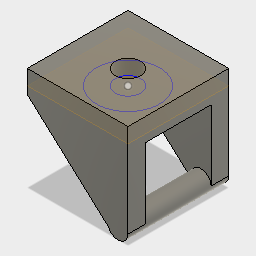
CasterWheelAngle (Autodesk Fusion 360 design; units mm, degrees)
Autodesk Fusion 360 part; units mm, degrees
sketch "Sketch1" plane through (0, 0, 0) normal (0, 1, 0) x (1, 0, 0)
  line L0 (0, 0) -> (40, 0)
  line L1 (40, 0) -> (40, -40)
  line L2 (40, -40) -> (0, -40)
  line L3 (0, -40) -> (0, 0)
  dimension "d1" = 40
  dimension "d2" = 40
  constraint horizontal L0
  constraint vertical L1
  constraint horizontal L2
  constraint vertical L3
  constraint coincident L0.start L3.end
extrude "Extrude1" add sketch "Sketch1" along normal blind 25 makes body 1
extrude "Extrude2" cut 1 faces at (13.3333, 0, 13.3333) along direction (0, 1, 0) blind 24 on bodies 1 bodies 1
extrude "Extrude3" add 1 faces at (13.3333, 25, 13.3333) along direction (0, 1, 0) blind 35 on bodies 1 bodies 1
extrude "Extrude4" add 1 faces at (13.3333, 24, 13.3333) along direction (0, -1, 0) blind 1 on bodies 1 bodies 1
extrude "Extrude5" cut 1 faces at (13.3333, 23, 13.3333) along direction (0, 1, 0) blind 2 on bodies 1 bodies 1
sketch "Sketch2" plane through (0, 0, 40) normal (0, 0, 1) x (1, 0, 0)
  line L0 (0, 25) -> (40, 25)
  line L1 (40, 25) -> (40, 60)
  line L2 (40, 60) -> (0, 60)
  line L3 (0, 60) -> (0, 25)
  line L4 (0, 60) -> (0, 51)
  line L5 (40, 25) -> (36, 25)
  line L6 (36, 25) -> (36, 29)
  circle A0 centre (36, 29) radius 4
  dimension "d13" = 9
  dimension "d14" = 4
  dimension "d15" = 4
  dimension "d16" = 8
  measures "d13" distance of origin
  measures "d16" diameter of A0
extrude "Extrude6" cut sketch "Sketch2" against normal blind 59 contours L0 L1 L5 A0 bodies 1
sketch "Sketch3" plane through (0, 0, 40) normal (0, 0, 1) x (1, 0, 0)
  arc A0 (36, 25) -> (40, 29) centre (36, 29) ccw
  line L0 (40, 29) -> (40, 60)
  line L1 (40, 60) -> (0, 60)
  line L2 (0, 60) -> (0, 25)
  line L3 (0, 25) -> (36, 25)
  line L4 (36, 25) -> (0, 50)
  constraint coincident L2 origin
extrude "Extrude7" cut sketch "Sketch3" against normal blind 192 contours L2 L3 L4 bodies 1
sketch "Sketch4" plane through (0, 0, 40) normal (0, 0, 1) x (1, 0, 0)
  line L0 (0, 50) -> (36, 25)
  arc A0 (36, 25) -> (40, 29) centre (36, 29) ccw
  line L1 (40, 29) -> (40, 60)
  line L2 (40, 60) -> (0, 60)
  line L3 (0, 60) -> (0, 50)
  line L4 (36, 25) -> (36, 29)
  circle A1 centre (36, 29) radius 4
  dimension "d21" = 4
  dimension "d22" = 8
  measures "d22" diameter of A1
extrude "Extrude8" add sketch "Sketch4" against normal blind 40 contours L0 A1 bodies 1
sketch "Sketch5" plane through (40, 0, 0) normal (1, 0, 0) x (0, 0, -1)
  line L0 (-40, 29) -> (0, 29)
  line L1 (0, 29) -> (0, 60)
  line L2 (0, 60) -> (-40, 60)
  line L3 (-40, 60) -> (-40, 29)
  line L4 (0, 60) -> (0, 51)
  line L5 (0, 51) -> (-7, 51)
  line L6 (-40, 51) -> (-33, 51)
  line L7 (-33, 51) -> (-33, 22)
  line L8 (-33, 22) -> (-7, 22)
  line L9 (-7, 22) -> (-7, 51)
  line L10 (-33, 51) -> (-7, 51)
  dimension "d25" = 9
  dimension "d26" = 7
  dimension "d27" = 7
  constraint vertical L4
  constraint coincident L3
  constraint perpendicular L0 L7
  constraint perpendicular L7 L8
  constraint perpendicular L5 L9
  constraint perpendicular L9 L10
  measures "d25" distance of origin
extrude "Extrude9" cut sketch "Sketch5" against normal blind 52 contours L0 L7 L9 L10 | L0 L7 L8 L9 bodies 1
sketch "Sketch6" plane through (0, 0, 33) normal (0, 0, -1) x (-1, 0, 0)
  arc A0 (-40, 29) -> (-32.252, 27.6028) centre (-36, 29) ccw
  line L0 (-32.252, 27.6028) -> (0, 50)
  line L1 (0, 50) -> (0, 51)
  line L2 (0, 51) -> (-40, 51)
  line L3 (-40, 51) -> (-40, 29)
  line L4 (-40, 29) -> (-36, 29)
  circle A1 centre (-36, 29) radius 4
  circle A2 centre (-36, 29) radius 4
  dimension "d30" = 4
  dimension "d31" = 8
  dimension "d32" = 8
  constraint concentric A1 A2
  measures "d31" diameter of A1
  measures "d32" diameter of A2
extrude "Extrude10" add sketch "Sketch6" against normal blind 7 separate body contours A0 A1 A2 makes body 2
sketch "Sketch7" plane through (0, 0, 7) normal (0, 0, 1) x (1, 0, 0)
  arc A0 (32.252, 27.6028) -> (40, 29) centre (36, 29) ccw
  line L0 (40, 29) -> (40, 51)
  line L1 (40, 51) -> (0, 51)
  line L2 (0, 51) -> (0, 50)
  line L3 (0, 50) -> (32.252, 27.6028)
  circle A1 centre (36, 29) radius 4
  dimension "d35" = 8
  constraint concentric A0 A1
  measures "d35" diameter of A1
extrude "Extrude11" add sketch "Sketch7" against normal blind 7 separate body contours A0 A1 makes body 3
sketch "Sketch8" plane through (0, 60, 0) normal (0, 1, 0) x (-1, 0, 0)
  line L0 (0, 40) -> (-40, 40)
  line L1 (-40, 40) -> (-40, 0)
  line L2 (-40, 0) -> (0, 0)
  line L3 (0, 0) -> (0, 40)
  circle A0 centre (-20, 20) radius 12.5
  circle A1 centre (-20, 20) radius 5
  dimension "d38" = 25
  dimension "d39" = 10
  constraint concentric A0 A1
  measures "d38" diameter of A0
  measures "d39" diameter of A1
extrude "Extrude12" cut sketch "Sketch8" against normal blind 1203 contours A1 bodies 1
extrude "Extrude13" cut sketch "Sketch8" against normal blind 2 contours A0 bodies 1
extrude "Extrude14" add 1 faces at (10.0652, 58, 19.1306) along direction (0, 1, 0) blind 2 on bodies 1 bodies 1
sketch "Sketch9" plane through (0, 51, 0) normal (0, -1, 0) x (1, 0, 0)
  circle A0 centre (20, 20) radius 5
  line L0 (0, 33) -> (0, 7)
  line L1 (0, 7) -> (40, 7)
  line L2 (40, 7) -> (40, 33)
  line L3 (40, 33) -> (0, 33)
  circle A1 centre (20, 20) radius 12.5
  dimension "d46" = 25
  constraint concentric A0 A1
  measures "d46" diameter of A1
extrude "Extrude15" cut sketch "Sketch9" against normal blind 2 contours A1 bodies 1
extrude "Extrude16" add 1 faces at (37.2498, 28.7186, 7) along direction (0, 0, 1) blind 26 separate body on bodies 3 makes body 4
extrude "Extrude17" cut 1 faces at (2.5, 51, 20) along direction (0, 1, 0) blind 4 on bodies 1 bodies 1
extrude "Extrude18" cut 1 faces at (29.9348, 53, 19.1306) along direction (0, 1, 0) blind 6 on bodies 1 bodies 1
extrude "Extrude19" add sketch "Sketch8" along normal blind 4 contours L0 L1 L2 L3 | A0 bodies 1
extrude "Extrude20" cut 1 faces at (2.5, 55, 20) along direction (0, 1, 0) blind 2 on bodies 1 bodies 1
extrude "Extrude21" add 1 faces at (19.8754, 64, 5.0047) along direction (0, 1, 0) blind 2 on bodies 1 bodies 1
sketch "Sketch10" plane through (0, 0, 40) normal (0, 0, 1) x (1, 0, 0)
  line L0 (0, 50) -> (32.252, 27.6028)
  arc A0 (32.252, 27.6028) -> (40, 29) centre (36, 29) ccw
  line L1 (40, 29) -> (40, 66)
  line L2 (40, 66) -> (0, 66)
  line L3 (0, 66) -> (0, 50)
  line L4 (0, 57) -> (32.252, 27.6028)
extrude "Extrude22" cut sketch "Sketch10" against normal blind 293 contours L0 L3 L4 bodies 1
extrude "Extrude23" add 1 faces at (34.9835, 28.3914, 40) along direction (0, 0, 1) blind 1 on bodies 2 bodies 2 3 4 1
extrude "Extrude24" cut 1 faces at (34.9835, 28.3914, 41) along direction (0, 0, -1) blind 1 on bodies 2 bodies 2
extrude "Extrude25" cut 1 faces at (37.2498, 28.7186, 0) along direction (0, 0, 1) blind 39 on bodies 3 bodies 2 3 4
extrude "Extrude26" add 1 faces at (37.2498, 28.7186, 39) along direction (0, 0, -1) blind 39 on bodies 2 bodies 2 3 4
copy_body "Body->Comp1" bodies 2 removing the originals makes body 5 in component "CasterWheelAngle"
component "CasterWheelAngle" placed x (1, 0, 0) y (0, 1, 0) z (0, 0, 1) at (0, 0, 0)
named bodies: "CasterWheelAngle"
